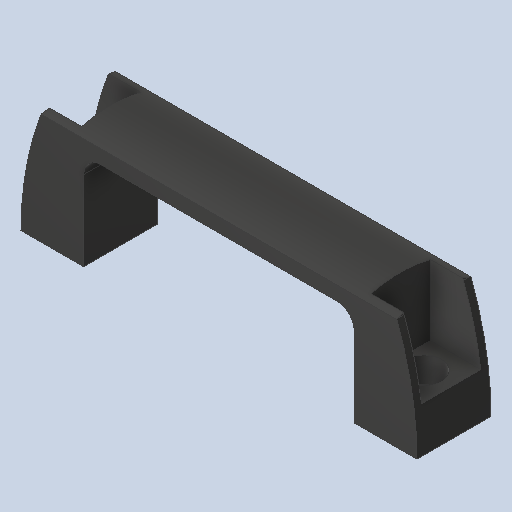
# Autodesk Inventor part: UPCN26-B-41
Saved by Autodesk Inventor 2024.2 (Build 282272000, 272)
## iProperties
Category: PARTsolutions
Company: MISUMI
Created: 2024-01-11
Part Number: UPCN26-B-41
Material: Generic
Description: UPCN_body-Handles - Non-Metal Type
Vendor: MISUMI
Document SubType Name: Modeling
Designer: psAdmin
Manufacturer: MISUMI
Mass: 37.8288 g
Surface Area: 172.479 cm^2
Volume: 37.8288 cm^3
Density: 1 g/cm^3
Appearance: Smooth - Black
Catalog Web Link: https://jp.misumi-ec.com/vona2/detail/110302239150/?ProductCode=UPCN26-B-41
PSOL_IDENT_0: {$CADENAS_DATA/23d-libs/misumi/metric/44_handles_hinges/upcn.prj},192 {VTYP=3D},{NB=UPCN26-B-41_b},{
PSOL_IDENT_1: LINA=UPCN26-B-41},{NN=UPCN_body},{DATE=29.05.2023 08:48:12},{GEOMDATE=15.11.2019 02:05:13},{VERSION=
PSOL_IDENT_2: },{LINEID=20},{WBVAR=COLORSE,COLOR,HSE,H,ALT1},{WBNUMERIC=H}  {NB=UPCN26-B-41_b},{LINA=UPCN26-B-41},
PSOL_IDENT_3: {KT=DUMMY},{PN=UPCN26-B-41},{MAT=Glass Fiber Reinforced Nylon 6 },{A=26},{COLORSE=COLSE},{COLORSEALG=''
PSOL_IDENT_4: ,'Not Specified','COLSE','Specified'},{COLOR=B},{COLORALG= 'B','Black','W','White','M','Orange','R','
PSOL_IDENT_5: Red','G','Green' },{COLORPN=-B},{HSE=HSE},{HSEALG='','Not Specified','HSE','Specified'},{H=41},{H1=[
PSOL_IDENT_6: 41,57]},{HPN=-41},{HH=34},{L=117.0},{L1=139.0},{R=8.5},{C=13.3},{LRR=15},{LCC=9},{AL=500},{MASS=38},
PSOL_IDENT_7: {ALT1=},{NO=8},{ALT1M=8},{ALT1M1=8},{ALT1BL=15},{ALT1BT=},{ALT1NT=},{ALT1NMAT=},{COLORC=0.00,0.00,0.
PSOL_IDENT_8: 00},{NUTCP=5.500}
NB: UPCN26-B-41_b
NN: UPCN_body
NT: Handles - Non-Metal Type
NBSYN: $PN._b
LINA: UPCN26-B-41
CATALOG: Misumi
PN: UPCN26-B-41
MAT: Glass Fiber Reinforced Nylon 6
A: 26
COLORSE: Specified
COLOR: Black
HSE: Specified
H: 41
HH: 34
L: 117
L1: 139
R: 8.5
C: 13.3
LRR: 15
LCC: 9
AL: 500
MASS: 38
ALT1: w/o Set of Applicable Bolt and Nut
NO: 8
SUPPLIER: MISUMI
ARTICLENO: UPCN26-B-41_b
BOMINFO: UPCN26-B-41
CREATOR: CADENAS GmbH
Title: UPCN26-B-41
Author: Cadenas PARTsolutions
Comments: Handles - Non-Metal Type
Autodesk Inventor part; units mm, degrees
sketch "Sketch_1" plane through (0, 0, 0) normal (0, 0, 1) x (1, 0, 0)
  line L0 (-11, 0) -> (11, 0)
  line L1 (11, 0) -> (11, 28)
  arc A0 (17, 34) -> (11, 28) centre (17, 28) ccw
  line L2 (17, 34) -> (100, 34)
  arc A1 (106, 28) -> (100, 34) centre (100, 28) ccw
  line L3 (106, 28) -> (106, 0)
  line L4 (106, 0) -> (128, 0)
  arc A2 (128, 0) -> (120.8624, 39.061) centre (17.55, 0) ccw
  arc A3 (120.8624, 39.061) -> (118.0562, 41) centre (118.0562, 38) ccw
  line L5 (118.0562, 41) -> (-1.0562, 41)
  arc A4 (-1.0562, 41) -> (-3.8624, 39.061) centre (-1.0562, 38) ccw
  arc A5 (-3.8624, 39.061) -> (-11, 0) centre (99.45, 0) ccw
  constraints: 12 end point, 12 point on circle, 6 centre point
extrude "Extrusion1" add sketch "Sketch_1" along normal mid plane 26
sketch "Sketch_2" plane through (0, 15, 0) normal (0, 1, 0) x (1, 0, 0)
  line L0 (-58.5, -26) -> (175.5, -26)
  line L1 (175.5, -26) -> (175.5, 26)
  line L2 (175.5, 26) -> (-58.5, 26)
  line L3 (-58.5, 26) -> (-58.5, -26)
  line L4 (-11, 10.4) -> (7.7, 10.4)
  line L5 (7.7, 10.4) -> (7.7, -10.4)
  line L6 (7.7, -10.4) -> (-11, -10.4)
  line L7 (-11, -10.4) -> (-11, -13)
  line L8 (-11, -13) -> (128, -13)
  line L9 (128, -13) -> (128, -10.4)
  line L10 (128, -10.4) -> (109.3, -10.4)
  line L11 (109.3, -10.4) -> (109.3, 10.4)
  line L12 (109.3, 10.4) -> (128, 10.4)
  line L13 (128, 10.4) -> (128, 13)
  line L14 (128, 13) -> (-11, 13)
  line L15 (-11, 13) -> (-11, 10.4)
  constraints: 32 end point
extrude "Extrusion2" cut sketch "Sketch_2" along normal blind 58.5
sketch "Sketch3" plane through (0, 15, 0) normal (0, 1, 0) x (1, 0, 0)
  point P0 (0, 0)
hole "Hole1" at (0, 15, 0) direction (0, -1, 0) diameter 8.5 depth 15 counterbore diameter 13.3 counterbore depth 9
sketch "Sketch4" plane through (0, 15, 0) normal (0, 1, 0) x (1, 0, 0)
  point P0 (117, 0)
hole "Hole2" at (117, 15, 0) direction (0, -1, 0) diameter 8.5 depth 15 counterbore diameter 13.3 counterbore depth 9
sketch "Sketch_6" plane through (-11, 0, 0) normal (1, 0, 0) x (0, 0, -1)
  line L0 (-13, 46) -> (-13, 38.8844)
  arc A0 (13, 38.8844) -> (-13, 38.8844) centre (0, 0) ccw
  line L1 (13, 38.8844) -> (13, 46)
  line L2 (13, 46) -> (-13, 46)
  constraints: 6 end point, 2 point on circle, 1 centre point
extrude "Extrusion3" cut sketch "Sketch_6" along normal blind 139
ref_plane "handle_to_body_XY" through (58.5, 0, 0) normal (0, 1, 0) x (1, 0, 0)
ref_plane "handle_to_body_YZ" through (58.5, 0, 0) normal (1, 0, 0) x (0, 0, -1)
ref_plane "handle_to_body_ZX" through (58.5, 0, 0) normal (0, 0, -1) x (0, 1, 0)
ref_plane "handle_to_bolt1_XY" through (117, 6, 0) normal (0, 1, 0) x (1, 0, 0)
ref_plane "handle_to_bolt1_YZ" through (117, 6, 0) normal (1, 0, 0) x (0, 0, -1)
ref_plane "handle_to_bolt1_ZX" through (117, 6, 0) normal (0, 0, -1) x (0, 1, 0)
ref_plane "handle_to_bolt2_XY" through (0, 6, 0) normal (0, 1, 0) x (1, 0, 0)
ref_plane "handle_to_bolt2_YZ" through (0, 6, 0) normal (1, 0, 0) x (0, 0, -1)
ref_plane "handle_to_bolt2_ZX" through (0, 6, 0) normal (0, 0, -1) x (0, 1, 0)
ref_plane "handle_to_nut1_XY" through (117, 0, 0) normal (0, 1, 0) x (1, 0, 0)
ref_plane "handle_to_nut1_YZ" through (117, 0, 0) normal (1, 0, 0) x (0, 0, -1)
ref_plane "handle_to_nut1_ZX" through (117, 0, 0) normal (0, 0, -1) x (0, 1, 0)
ref_plane "handle_to_nut2_XY" through (0, 0, 0) normal (0, 1, 0) x (1, 0, 0)
ref_plane "handle_to_nut2_YZ" through (0, 0, 0) normal (1, 0, 0) x (0, 0, -1)
ref_plane "handle_to_nut2_ZX" through (0, 0, 0) normal (0, 0, -1) x (0, 1, 0)
ref_plane "to_nut_1_XY" through (0, -5.5, 0) normal (0, -1, 0) x (1, 0, 0)
ref_plane "to_nut_1_YZ" through (0, -5.5, 0) normal (1, 0, 0) x (0, 0, 1)
ref_plane "to_nut_1_ZX" through (0, -5.5, 0) normal (0, 0, 1) x (0, -1, 0)
ref_plane "to_nut_2_XY" through (117, -5.5, 0) normal (0, -1, 0) x (1, 0, 0)
ref_plane "to_nut_2_YZ" through (117, -5.5, 0) normal (1, 0, 0) x (0, 0, 1)
ref_plane "to_nut_2_ZX" through (117, -5.5, 0) normal (0, 0, 1) x (0, -1, 0)
body "Solid1"
